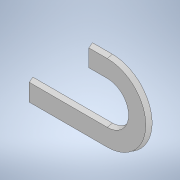
# Autodesk Inventor part: hook
Saved by Autodesk Inventor 2020 (Build 240168000, 168)
## iProperties
Created: 2020-01-24
Part Number: hook
Material: Generic
Document SubType Name: Modeling
Designer: 1sfkeith
Density: 1 g/cm^3
Appearance: Default
Author: 1sfkeith
Autodesk Inventor part; units mm, degrees
ref_plane "YZ Plane" through (0, 0, 0) normal (1, 0, 0) x (0, 1, 0)
ref_plane "XZ Plane" through (0, 0, 0) normal (0, 1, 0) x (-1, 0, 0)
ref_plane "XY Plane" through (0, 0, 0) normal (0, 0, 1) x (1, 0, 0)
sketch "Sketch1" plane through (0, 0, 0) normal (0, 0, 1) x (1, 0, 0)
  line L0 (198.6992, 316.0095) -> (224.0992, 316.0095)
  line L1 (274.8992, 265.2095) -> (274.8992, 265.2095)
  line L2 (224.0992, 214.4095) -> (122.4992, 214.4095)
  line L3 (198.4116, 290.6095) -> (224.0992, 290.6095)
  line L4 (249.4992, 265.2095) -> (249.4992, 265.2095)
  line L5 (224.0992, 239.8095) -> (122.4992, 239.8095)
  line L6 (198.6992, 316.0095) -> (198.6992, 290.6095)
  line L7 (122.4992, 239.8095) -> (122.4992, 214.4095)
  arc A0 (249.4992, 265.2095) -> (224.0992, 290.6095) centre (224.0992, 265.2095) ccw
  arc A1 (224.0992, 239.8095) -> (249.4992, 265.2095) centre (224.0992, 265.2095) ccw
  arc A2 (274.8992, 265.2095) -> (224.0992, 316.0095) centre (224.0992, 265.2095) ccw
  arc A3 (224.0992, 214.4095) -> (274.8992, 265.2095) centre (224.0992, 265.2095) ccw
  point P0 (0, 0)
  point P1 (274.8992, 316.0095)
  point P2 (274.8992, 214.4095)
  dimension "d0" = 50.8
  dimension "d1" = 25.4
  dimension "d2" = 25.4
  dimension "d3" = 25.4
  dimension "d4" = 76.2
  dimension "d5" = 25.4
  dimension "d6" = 152.4
  dimension "d7" = 25.4
  dimension "d8" = 25.4
  dimension "d9" = 50.8
  constraints: 16 end point, 8 point on circle, 8 tangent, 5 point on line, 4 centre point, 4 horizontal, 1 concentric, 1 vertical
  measures "d0" distance between parallel lines of L5 L3
  measures "d1" distance between parallel lines of L3 L0
  measures "d2" distance between parallel lines of L2 L5
  measures "d3" distance between parallel lines of L1 L4
  measures "d4" distance of L0.start point (274.899, 316.01)
  measures "d5" distance of L5.end L2.end
  measures "d6" distance of point (274.899, 214.41) L2.end
  measures "d7" radius of A0
  measures "d8" radius of A1
  measures "d9" radius of A2
extrude "Extrusion1" add sketch "Sketch1" along normal blind 6.35 draft -15
body "Solid1"
